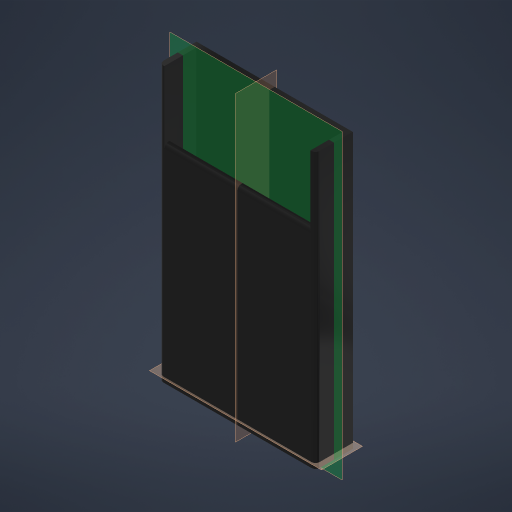
# Autodesk Inventor part: Powerbank Holder
Saved by Autodesk Inventor 2024 (Build 280153000, 153)
## iProperties
Manager: Louis Van Roosmaelen
Company: DCS - DIGITAL COMBAT SIMULATOR
Created: 2023-11-01
Part Number: Powerbank Holder
Material: S235
Catalog Web Link: http://emmausbovenbouw.op-weg.be/
Vendor: Emmaüsinstituut Bovenbouw Aalter
Document SubType Name: Modeling
Designer: Louis
Engineer: Declercq St.
Manufacturer: Standard
Standards Organization: Custom
Density: 7.86 g/cm^3
Appearance: Smooth - Black
IDENT.NR.: AJ2022
TEAM: 30
Title: F18C Home Cockpit
Author: Louis
Keywords: Ø
Autodesk Inventor part; units mm, degrees
sketch "Sketch1" plane through (0, 0, 0) normal (0, 0, 1) x (1, 0, 0)
  line L0 (0, 2.8582) -> (0, -2.8582) construction
  line L1 (-5.7775, 0) -> (5.7775, 0) construction
  line L2 (-35.25, -6.5) -> (35.25, -6.5)
  line L3 (35.25, -6.5) -> (35.25, 6.5)
  line L4 (35.25, 6.5) -> (-35.25, 6.5)
  line L5 (-35.25, 6.5) -> (-35.25, -6.5)
  line L6 (-35.25, -6.5) -> (35.25, 6.5) construction
  line L7 (35.25, -6.5) -> (-35.25, 6.5) construction
  line L8 (-37.75, 9) -> (37.75, 9)
  line L9 (37.75, 9) -> (37.75, -9)
  line L10 (37.75, -9) -> (-37.75, -9)
  line L11 (-37.75, -9) -> (-37.75, 9)
  line L12 (-37.75, 9) -> (37.75, -9) construction
  line L13 (37.75, 9) -> (-37.75, -9) construction
  point P0 (0, 0)
  point P1 (0, 0)
  dimension "d0" = 70.5
  dimension "d1" = 13
  dimension "d2" = 2.5
  dimension "d3" = 2.5
  constraints: 28 end point, 6 midpoint, 4 parallel, 3 horizontal, 2 perpendicular, 1 coincident, 1 vertical
  measures "d0" distance of L4.end L3.end
  measures "d1" distance of L3.end L2.end
  measures "d2" distance between parallel lines of L11 L5
  measures "d3" distance between parallel lines of L4 L8
extrude "Extrusion1" add sketch "Sketch1" along normal blind 130
sketch "Sketch2" plane through (0, 0, 0) normal (0, 0, -1) x (-1, 0, 0)
  line L0 (-35.25, -6.5) -> (35.25, -6.5) projected
  line L1 (35.25, -6.5) -> (35.25, 6.5) projected
  line L2 (35.25, 6.5) -> (-35.25, 6.5) projected
  line L3 (-35.25, 6.5) -> (-35.25, -6.5) projected
  line L4 (37.75, 9) -> (37.75, -9) projected
  line L5 (37.75, -9) -> (-37.75, -9) projected
  line L6 (-37.75, -9) -> (-37.75, 9) projected
  line L7 (-37.75, 9) -> (37.75, 9) projected
  point P0 (0, 0)
extrude "Extrusion2" add sketch "Sketch2" along normal blind 2.5 contours L3 L2 L1 L0 | L4 L5 L6 L7
sketch "Sketch3" plane through (-37.75, -9, 130) normal (0, -1, 0) x (1, 0, 0)
  line L0 (75.5, -132.5) -> (0, -132.5) projected
  line L1 (0, -132.5) -> (0, 0) projected
  line L2 (0, 0) -> (75.5, 0) projected
  line L3 (75.5, 0) -> (75.5, -132.5) projected
  line L4 (0, -32.5) -> (75.5, -32.5)
  line L5 (2.5, -130) -> (2.5, 0) projected
  line L6 (73, -130) -> (73, 0) projected
  point P0 (37.75, -130)
  point P1 (73, -32.5)
  point P2 (2.5, -32.5)
  dimension "d8" = 100
  constraints: 2 end point, 2 point on line, 1 perpendicular
  measures "d8" distance between parallel lines of L0 L4
extrude "Extrusion3" cut sketch "Sketch3" against normal up to surface (2.5 mm away) contours L4 L5 L2 L6
fillet "Fillet1" radius 2 1 edges at (0, -9, 97.5)
fillet "Fillet2" radius 2 2 edges at (-37.75, -9, 63.75) (37.75, -9, 63.75)
equation "\"d3\" = d2"
body "Solid1"
